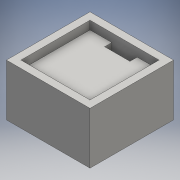
# Autodesk Inventor part: Pantalla
Saved by Autodesk Inventor 2016 (Build 200138000, 138)
## iProperties
Created: 2016-04-24
Part Number: Pantalla
Material: Generic
Document SubType Name: Modeling
Designer: Freddy Chang
Density: 1 g/cm^3
Appearance: Default
Author: Freddy Chang
Autodesk Inventor part; units mm, degrees
ref_plane "YZ Plane" through (0, 0, 0) normal (1, 0, 0) x (0, 1, 0)
ref_plane "XZ Plane" through (0, 0, 0) normal (0, 1, 0) x (-1, 0, 0)
ref_plane "XY Plane" through (0, 0, 0) normal (0, 0, 1) x (1, 0, 0)
sketch "Sketch1" plane through (0, 0, 0) normal (0, 0, 1) x (1, 0, 0)
  line L0 (0, 0) -> (34.66, 0)
  line L1 (34.66, 0) -> (34.66, -34.66)
  line L2 (34.66, -34.66) -> (0, -34.66)
  line L3 (0, -34.66) -> (0, 0)
  dimension "d0" = 34.66
  dimension "d1" = 34.66
  constraints: 8 end point, 2 parallel, 1 horizontal, 1 perpendicular
  measures "d0" distance of L1.end L2.end
  measures "d1" distance of L0.end L1.end
extrude "Extrusion1" add sketch "Sketch1" along normal blind 21.5
sketch "Sketch2" plane through (0, 0, 21.5) normal (0, 0, 1) x (1, 0, 0)
  line L0 (0, 0) -> (0, -34.66) projected
  line L1 (3, -3) -> (31.66, -3)
  line L2 (31.66, -3) -> (31.66, -31.66)
  line L3 (31.66, -31.66) -> (3, -31.66)
  line L4 (3, -31.66) -> (3, -3)
  line L5 (34.66, 0) -> (0, 0) projected
  line L6 (0, -34.66) -> (34.66, -34.66) projected
  line L7 (34.66, 0) -> (34.66, -34.66) projected
  dimension "d8" = 3
  dimension "d9" = 3
  dimension "d10" = 3
  dimension "d11" = 3
  constraints: 8 end point, 2 parallel, 1 horizontal, 1 perpendicular
  measures "d8" distance between parallel lines of L5 L1
  measures "d9" distance between parallel lines of L6 L3
  measures "d10" distance between parallel lines of L7 L2
  measures "d11" distance between parallel lines of L0 L4
extrude "Extrusion2" cut sketch "Sketch2" against normal blind 3.5 contours L1 L2 L3 L4
sketch "Sketch3" plane through (0, 0, 18) normal (0, 0, 1) x (1, 0, 0)
  line L0 (12.08, -3) -> (12.08, -6)
  line L1 (12.08, -6) -> (22.58, -6)
  line L2 (22.58, -6) -> (22.58, -3)
  line L3 (12.08, -3) -> (22.58, -3)
  line L4 (3, -3) -> (31.66, -3) projected
  line L5 (3, -31.66) -> (3, -3) projected
  line L6 (31.66, -3) -> (31.66, -31.66) projected
  line L7 (31.66, -31.66) -> (3, -31.66) projected
  point P0 (0, 0)
  dimension "d18" = 9.08
  dimension "d19" = 9.08
  dimension "d20" = 3
  dimension "d21" = 28.66
  constraints: 8 end point, 1 collinear, 1 horizontal, 1 perpendicular, 1 vertical
  measures "d18" distance between parallel lines of L5 L0
  measures "d19" distance between parallel lines of L6 L2
  measures "d20" distance between parallel lines of L3 L1
  measures "d21" distance between parallel lines of L3 L7
extrude "Extrusion3" cut sketch "Sketch3" against normal blind 19 contours L3 L2 L1 L0
body "Solid1"
